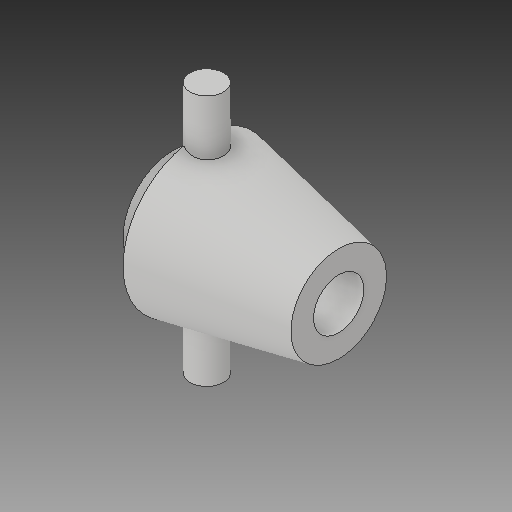
# Autodesk Inventor part: Arm_Wheel_Attachment
Saved by Autodesk Inventor 2019 (Build 230136000, 136)
## iProperties
Created: 2019-03-03
Part Number: Arm_Wheel_Attachment
Material: Generic
Document SubType Name: Modeling
Designer: alarr
Density: 1 g/cm^3
Appearance: Default
Author: alarr
Autodesk Inventor part; units mm, degrees
ref_plane "YZ Plane" through (0, 0, 0) normal (1, 0, 0) x (0, 1, 0)
ref_plane "XZ Plane" through (0, 0, 0) normal (0, 1, 0) x (-1, 0, 0)
ref_plane "XY Plane" through (0, 0, 0) normal (0, 0, 1) x (1, 0, 0)
sketch "Sketch1" plane through (0, 0, 0) normal (0, 0, 1) x (1, 0, 0)
  line L0 (87.63, 0) -> (112.6819, 0)
  line L1 (112.6819, 0) -> (112.6819, 7.239)
  line L2 (112.6819, 7.239) -> (91.44, 11.43)
  line L3 (87.63, 11.43) -> (87.63, 7.62) construction
  line L4 (85.09, -8.9952) -> (85.09, 8.9952) projected
  line L5 (85.09, 0) -> (87.63, 0) construction
  arc A0 (91.44, 11.43) -> (87.63, 7.62) centre (87.63, 11.43) ccw construction
  arc A1 (87.63, 7.62) -> (91.44, 11.43) centre (87.63, 11.43) ccw
  line L6 (87.63, 7.62) -> (87.63, 0)
  line L7 (91.44, 11.43) -> (87.63, 11.43) construction
  point P0 (0, 0)
  dimension "d0" = 25.4
  dimension "d1" = 11.43
  dimension "d2" = 2.54
  dimension "d3" = 7.62
  dimension "d5" = 7.239
  constraints: 14 end point, 4 point on circle, 3 parallel, 2 centre point, 2 horizontal, 1 coincident, 1 midpoint, 1 perpendicular
  measures "d0" distance of L1.end L3.start
  measures "d1" distance of L3.start L0.start
  measures "d2" distance between parallel lines of L3 L4
  measures "d3" diameter of A0
  measures "d5" distance of L0.end L1.end
revolve "Revolution1" add sketch "Sketch1" angle 360 about axis through (87.63, 0, 0) along (1, 0, 0)
sketch "Sketch2" plane through (0, 0, 0) normal (0, 1, 0) x (-1, 0, 0)
  circle A0 centre (-92.71, 0) radius 2.54 projected
  circle A1 centre (-92.71, 0) radius 2.54 projected
  circle A2 centre (-92.71, 0) radius 2.54 projected
  circle A3 centre (-92.71, 0) radius 2.54 projected
  circle A4 centre (-92.71, 0) radius 2.54
  point P0 (0, 0)
  constraints: 1 centre point, 1 coincident, 1 concentric
extrude "Extrusion1" add sketch "Sketch2" along normal mid plane 38.1
sketch "Sketch3" plane through (112.6819, 0, 0) normal (1, 0, 0) x (0, 0, -1)
  circle A0 centre (0, 0) radius 3.81
  dimension "d8" = 7.62
  constraints: 1 centre point, 1 coincident
  measures "d8" diameter of A0
extrude "Extrusion2" cut sketch "Sketch3" against normal blind 12.7
body "Solid1"
